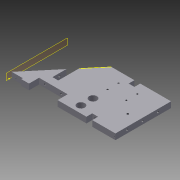
# Autodesk Inventor part: Chassis Right3
Saved by Autodesk Inventor 2012 (Build 160160000, 160)
## iProperties
Created: 2012-04-02
Part Number: Chassis Right3
Material: Aluminum-6061
Document SubType Name: Modeling
Designer: Jaime
Density: 2.71 g/cm^3
Mass: 278.782 g
Surface Area: 303.052 cm^2
Volume: 102.872 cm^3
Author: Jaime
Autodesk Inventor part; units mm, degrees
ref_plane "YZ Plane" through (0, 0, 0) normal (1, 0, 0) x (0, 1, 0)
ref_plane "XZ Plane" through (0, 0, 0) normal (0, 1, 0) x (-1, 0, 0)
ref_plane "XY Plane" through (0, 0, 0) normal (0, 0, 1) x (1, 0, 0)
sketch "Sketch1" plane through (0, 0, 0) normal (0, 0, 1) x (1, 0, 0)
  line L0 (0, 0) -> (175, 0)
  line L1 (175, 0) -> (175, 91.44)
  line L2 (175, 91.44) -> (76.7273, 91.44)
  line L3 (76.7273, 91.44) -> (0, 0)
  dimension "d0" = 175
  dimension "d1" = 91.44
  dimension "d100" = 50
  constraints: 8 end point, 1 horizontal, 1 parallel, 1 perpendicular
  measures "d0" distance of L0.start L0.end
  measures "d1" distance of L0.end L1.end
  measures "d100" angle of L0 L3
extrude "Extrusion1" add sketch "Sketch1" along normal blind 9.525
sketch "Sketch8" plane through (0, 0, 0) normal (0, 0, -1) x (-1, 0, 0)
  circle A0 centre (-106.6758, 31.4833) radius 6.35 projected
  circle A1 centre (-106.6758, 11.5887) radius 6.35 projected
  dimension "d101" = 12.7
  dimension "d102" = 12.7
  measures "d101" diameter of A0
  measures "d102" diameter of A1
extrude "Extrusion2" cut sketch "Sketch8" against normal blind 25.4
sketch "Sketch9" plane through (0, 0, 0) normal (0, -1, 0) x (1, 0, 0)
  line L0 (175, 9.525) -> (0, 9.525) projected
  line L1 (0, 0) -> (0, 9.525) projected
  line L2 (0, 0) -> (175, 0) projected
  line L3 (33.02, 9.525) -> (80.01, 9.525)
  line L4 (80.01, 9.525) -> (80.01, 0)
  line L5 (80.01, 0) -> (33.02, 0)
  line L6 (33.02, 0) -> (33.02, 9.525)
  dimension "d105" = 33.02
  dimension "d106" = 46.99
  constraints: 8 end point, 2 parallel, 2 point on line, 1 horizontal, 1 perpendicular
  measures "d105" distance between parallel lines of L6 L1
  measures "d106" distance between parallel lines of L4 L6
extrude "Extrusion3" cut sketch "Sketch9" against normal blind 16.51 contours L4 L2 L6 L0
sketch "Sketch12" plane through (76.7273, 91.44, 0) normal (0, 1, 0) x (1, 0, 0)
  line L0 (-76.7273, -9.525) -> (0, -9.525) projected
  line L1 (0, 0) -> (0, -9.525) projected
  line L2 (0, 0) -> (-76.7273, 0) projected
  line L3 (-76.7273, 0) -> (-76.7273, -9.525) projected
  line L4 (-24.13, 0) -> (-33.655, 0)
  line L5 (-33.655, 0) -> (-33.655, -9.525)
  line L6 (-33.655, -9.525) -> (-24.13, -9.525)
  line L7 (-24.13, -9.525) -> (-24.13, 0)
  dimension "d109" = 24.13
  dimension "d110" = 9.525
  constraints: 8 end point, 2 parallel, 2 point on line, 1 horizontal, 1 perpendicular
  measures "d109" distance between parallel lines of L1 L7
  measures "d110" distance between parallel lines of L7 L5
extrude "Extrusion4" cut sketch "Sketch12" against normal blind 62.992 contours L5 L2 L7 L0
sketch "Sketch13" plane through (0, 0, 0) normal (0, -1, 0) x (1, 0, 0)
  line L0 (0, 0) -> (33.02, 0) projected
  line L1 (0, 9.525) -> (20.32, 9.525)
  line L2 (20.32, 9.525) -> (20.32, 0)
  line L3 (20.32, 0) -> (0, 0)
  line L4 (0, 0) -> (0, 9.525)
  dimension "d113" = 20.32
  constraints: 8 end point, 2 parallel, 1 horizontal, 1 perpendicular, 1 point on line
  measures "d113" distance between parallel lines of L2 L4
extrude "Extrusion5" cut sketch "Sketch13" against normal blind 2.54
sketch "Sketch14" plane through (76.7273, 91.44, 0) normal (0, 1, 0) x (1, 0, 0)
  line L0 (0, -9.525) -> (98.2727, -9.525) projected
  line L1 (98.2727, 0) -> (0, 0) projected
  line L2 (0, 0) -> (0, -9.525) projected
  line L3 (38.1, 0) -> (47.625, 0)
  line L4 (47.625, 0) -> (47.625, -9.525)
  line L5 (47.625, -9.525) -> (38.1, -9.525)
  line L6 (38.1, -9.525) -> (38.1, 0)
  point P0 (-76.7273, 0)
  dimension "d116" = 9.525
  dimension "d117" = 38.1
  constraints: 8 end point, 2 parallel, 2 point on line, 1 horizontal, 1 perpendicular
  measures "d116" distance between parallel lines of L4 L6
  measures "d117" distance between parallel lines of L2 L6
extrude "Extrusion6" cut sketch "Sketch14" against normal blind 9.525 contours L6 L1 L4 L0
sketch "Sketch15" plane through (175, 0, 0) normal (0, -1, 0) x (1, 0, 0)
  line L0 (-94.99, 0) -> (0, 0) projected
  line L1 (0, 0) -> (0, 9.525) projected
  line L2 (0, 9.525) -> (-94.99, 9.525) projected
  line L3 (-38.1, 9.525) -> (-47.625, 9.525)
  line L4 (-47.625, 9.525) -> (-47.625, 0)
  line L5 (-47.625, 0) -> (-38.1, 0)
  line L6 (-38.1, 0) -> (-38.1, 9.525)
  point P0 (-175, 0)
  dimension "d120" = 38.1
  dimension "d121" = 9.525
  constraints: 8 end point, 2 parallel, 2 point on line, 1 horizontal, 1 perpendicular
  measures "d120" distance between parallel lines of L1 L6
  measures "d121" distance between parallel lines of L6 L4
extrude "Extrusion7" cut sketch "Sketch15" against normal blind 9.525 contours L4 L2 L6 L0
sketch "Sketch16" plane through (76.7273, 81.915, 0) normal (0, 1, 0) x (1, 0, 0)
  circle A0 centre (42.8625, -4.7625) radius 2.2479 projected
  point P0 (-76.7273, 0)
  constraints: 1 coincident
hole "Hole7" at (119.5898, 81.915, 4.7625) direction (0, -1, 0) diameter 3.302 depth 10.16 tip angle 118 thread size "8-32 UNC" class "2B" standard "ANSI Unified Screw Threads"
sketch "Sketch17" plane through (175, 9.525, 0) normal (0, -1, 0) x (1, 0, 0)
  circle A0 centre (-42.8625, 4.7625) radius 2.2479 projected
  point P0 (-175, 0)
  constraints: 1 coincident
hole "Hole8" at (132.1375, 9.525, 4.7625) direction (0, 1, 0) diameter 3.302 depth 12.7 tip angle 118 thread size "8-32 UNC" class "2B" standard "ANSI Unified Screw Threads"
sketch "Sketch18" plane through (0, 16.51, 0) normal (0, -1, 0) x (1, 0, 0)
  circle A0 centre (42.5958, 4.7625) radius 2.2479 projected
  circle A1 centre (69.2658, 4.7625) radius 2.2479 projected
  point P0 (0, 0)
  constraints: 2 coincident
hole "Hole9" at (42.5958, 16.51, 4.7625) at (69.2658, 16.51, 4.7625) direction (0, 1, 0) diameter 3.302 depth 10.16 tip angle 118 thread size "8-32 UNC" class "2B" standard "ANSI Unified Screw Threads"
sketch "Sketch19" plane through (0, 0, 9.525) normal (0, 0, 1) x (1, 0, 0)
  circle A0 centre (105.912, 74.168) radius 1.8034 projected
  circle A1 centre (105.912, 56.134) radius 1.8034 projected
  circle A2 centre (136.9, 56.134) radius 1.8034 projected
  circle A3 centre (136.9, 74.168) radius 1.8034 projected
  point P0 (0, 0)
  constraints: 4 coincident
hole "Hole10" at (105.912, 74.168, 9.525) at (136.9, 74.168, 9.525) at (136.9, 56.134, 9.525) at (105.912, 56.134, 9.525) direction (0, 0, -1) diameter 2.6416 end through all thread size "6-32 UNC" class "2B" standard "ANSI Unified Screw Threads"
sketch "Sketch20" plane through (175, 0, 0) normal (1, 0, 0) x (0, 0, -1)
  line L0 (0, 0) -> (-9.525, 0) projected
  point P0 (-4.7625, 69.85)
  point P1 (-4.7625, 44.45)
  point P2 (-4.7625, 19.304)
  dimension "d152" = 19.304
  dimension "d153" = 44.45
  dimension "d154" = 69.85
  measures "d152" distance from line of L0 point (-4.763, 19.304)
  measures "d153" distance from line of L0 point (-4.763, 44.45)
  measures "d154" distance from line of L0 point (-4.763, 69.85)
hole "Hole11" at (175, 69.85, 4.7625) at (175, 44.45, 4.7625) at (175, 19.304, 4.7625) direction (-1, 0, 0) diameter 3.302 depth 12.7 tip angle 118 thread size "8-32 UNC" class "2B" standard "ANSI Unified Screw Threads"
sketch "Sketch21" plane through (43.0723, 51.3315, 0) normal (-0.7660444, 0.6427876, 0) x (0, 0, 1)
  circle A0 centre (4.7625, -32.4146) radius 2.2479 projected
  circle A1 centre (4.7625, 19.3379) radius 2.159 projected
  circle A2 centre (4.7625, 44.7379) radius 2.159 projected
  point P0 (0, -67.0086)
  constraints: 3 coincident
hole "Hole12" at (71.8292, 85.6027, 4.7625) at (55.5024, 66.1452, 4.7625) at (22.2366, 26.5005, 4.7625) direction (0.7660444, -0.6427876, 0) diameter 3.302 depth 7.62 tip angle 118 thread size "8-32 UNC" class "2B" standard "ANSI Unified Screw Threads"
sketch "Sketch22" plane through (43.0723, 51.3315, 0) normal (-0.7660444, 0.6427876, 0) x (0, 0, 1)
  circle A0 centre (4.7625, -53.0521) radius 2.159 projected
  point P0 (0, -67.0086)
  constraints: 1 coincident
hole "Hole13" at (8.971, 10.6913, 4.7625) direction (0.7660444, -0.6427876, 0) diameter 3.302 depth 7.62 tip angle 118 thread size "8-32 UNC" class "2B" standard "ANSI Unified Screw Threads"
sketch "Sketch23" plane through (0, 2.54, 0) normal (0, -1, 0) x (1, 0, 0)
  circle A0 centre (9.398, 3.81) radius 1.2192 projected
  point P0 (0, 0)
  constraints: 1 coincident
hole "Hole14" at (9.398, 2.54, 3.81) direction (0, 1, 0) diameter 1.7018 depth 2.54 tip angle 118
sketch "Sketch24" plane through (175, 0, 0) normal (0, -1, 0) x (1, 0, 0)
  circle A0 centre (-1.778, 3.81) radius 1.2192 projected
  point P0 (-175, 0)
  constraints: 1 coincident
hole "Hole15" at (173.222, 0, 3.81) direction (0, 1, 0) diameter 1.7018 depth 5.08 tip angle 118
ref_plane "Work Plane1" through (0, 0, 0) normal (1, 0, 0) x (0, 0, -1)
sketch "Sketch25" plane through (0, 0, 0) normal (1, 0, 0) x (0, 0, -1)
  circle A0 centre (-4.7625, 39.878) radius 2.159 projected
  point P0 (0, 0)
  constraints: 1 coincident
hole "Hole16" at (0, 39.878, 4.7625) direction (1, 0, 0) diameter 3.302 depth 76.2 tip angle 118 thread size "8-32 UNC" class "2B" standard "ANSI Unified Screw Threads"
sketch "Sketch26" plane through (0, 0, 9.525) normal (0, 0, 1) x (1, 0, 0)
  line L0 (139.44, 43.815) -> (175, 43.815) projected
  line L1 (175, 40.64) -> (175, 43.815) projected
  line L2 (139.44, 40.64) -> (175, 40.64) projected
  line L3 (139.44, 40.64) -> (139.44, 43.815) projected
  circle A0 centre (157.22, 37.9984) radius 2.4824
  point P0 (0, 0)
  dimension "d198" = 2.6416
  dimension "d199" = 4.9648
  constraints: 1 centre point, 1 coincident
  measures "d198" distance from line of L2 A0.centre
  measures "d199" diameter of A0
hole "Hole17" at (157.22, 37.9984, 9.525) direction (0, 0, -1) diameter 3.302 depth 4.7625 tip angle 118 thread size "8-32 UNC" class "2B" standard "ANSI Unified Screw Threads"
sketch "Sketch27" plane through (76.7273, 91.44, 0) normal (-0.7660444, 0.6427876, 0) x (0, 0, 1)
  circle A0 centre (4.7625, -33.02) radius 1.651 projected
  circle A1 centre (4.7625, -7.62) radius 1.651 projected
  line L0 (0, -37.5396) -> (9.525, -37.5396) projected
  line L1 (9.525, -37.5396) -> (9.525, 0) projected
  line L2 (0, 0) -> (9.525, 0) projected
  line L3 (0, 0) -> (0, -37.5396) projected
  point P0 (0, -119.3664)
body "Solid1"
